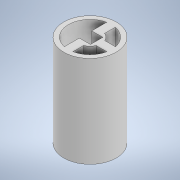
# Autodesk Inventor part: axel
Saved by Autodesk Inventor 2020 (Build 240168000, 168)
## iProperties
Created: 2019-10-28
Part Number: axel
Material: Generic
Document SubType Name: Modeling
Designer: dlr6513
Density: 1 g/cm^3
Appearance: Default
Author: dlr6513
Autodesk Inventor part; units mm, degrees
ref_plane "YZ Plane" through (0, 0, 0) normal (1, 0, 0) x (0, 1, 0)
ref_plane "XZ Plane" through (0, 0, 0) normal (0, 1, 0) x (-1, 0, 0)
ref_plane "XY Plane" through (0, 0, 0) normal (0, 0, 1) x (1, 0, 0)
sketch "Sketch1" plane through (0, 0, 0) normal (0, 1, 0) x (-1, 0, 0)
  circle A0 centre (0, 0) radius 20
  line L0 (-8.6, 0) -> (3.4, 0)
  line L1 (3.4, 0) -> (3.4, 7.8994)
  line L2 (3.4, 0) -> (3.4, -7.8994)
  line L3 (3.4, 0) -> (-5.1, 0)
  line L4 (-5.1, 0) -> (-5.1, -4.75)
  line L5 (-5.1, -4.75) -> (3.4, -4.75)
  line L6 (3.4, -4.75) -> (3.4, 0)
  line L7 (-5.1, 0) -> (-5.1, 4.75)
  line L8 (-5.1, 4.75) -> (3.4, 4.75)
  line L9 (-3.1555, 7.8994) -> (-3.1555, 16.1927)
  line L10 (-7.9441, -3.2941) -> (-16.1651, -3.2941)
  line L11 (3.1555, 19.7495) -> (3.4, 19.7495)
  line L12 (-3.1555, -7.8994) -> (-3.1555, -16.1927)
  line L13 (-7.9441, 3.2613) -> (-16.1717, 3.2613)
  line L14 (3.4, 19.7495) -> (3.4, 19.7089)
  line L15 (3.4, 16.1431) -> (3.4, 7.8994)
  line L16 (-8.6, -0.0164) -> (-7.9441, -0.0164)
  line L17 (3.4, -19.7495) -> (3.4, -19.7089)
  line L18 (3.4, -16.1431) -> (3.4, -7.8994)
  arc A1 (-7.9441, -3.2941) -> (-3.1555, -8.0002) centre (0, 0) ccw
  arc A2 (-3.1555, 8.0002) -> (-7.9576, 3.2613) centre (0, 0) ccw
  arc A3 (-8.6, 0) -> (-8.6, -0.0164) centre (0, 0) ccw
  arc A4 (3.4, -16.1431) -> (3.4, 16.1431) centre (0, 0) ccw
  arc A5 (-3.1555, 16.1927) -> (-16.1717, 3.2613) centre (0, 0) ccw
  arc A6 (-16.1651, -3.2941) -> (-3.1555, -16.1927) centre (0, 0) ccw
  point P0 (-3.1555, 19.7495)
  point P1 (-19.7269, -3.2941)
  point P2 (-3.1555, -19.7495)
  point P3 (-19.7269, 3.2613)
  dimension "d0" = 40
  dimension "d2" = 12
  dimension "d4" = 8.5
  constraints: 38 end point, 17 point on circle, 7 centre point, 5 parallel, 5 symmetric about line, 4 point on line, 3 coincident, 3 horizontal, 1 perpendicular, 1 vertical
  measures "d0" diameter of A0
  measures "d2" distance of L0.start L0.end
  measures "d4" distance between parallel lines of L4 L2
extrude "Extrusion1" add sketch "Sketch1" along normal blind 70 contours A0
equation "\"d6\" = 0.5 * d5"
equation "\"d5\" = 6.555455"
body "Solid1"
